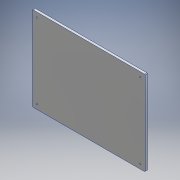
# Autodesk Inventor part: Breadboard
Saved by Autodesk Inventor 2016 (Build 200138000, 138)
## iProperties
Created: 2015-08-25
Part Number: Breadboard
Material: Aluminum 6061
Document SubType Name: Modeling
Designer: Conor Mow-Lowry
Density: 2.7 g/cm^3
Appearance: Aluminum - Flat
Author: Conor Mow-Lowry
Autodesk Inventor part; units mm, degrees
ref_plane "YZ Plane" through (0, 0, 0) normal (1, 0, 0) x (0, 1, 0)
ref_plane "XZ Plane" through (0, 0, 0) normal (0, 1, 0) x (-1, 0, 0)
ref_plane "XY Plane" through (0, 0, 0) normal (0, 0, 1) x (1, 0, 0)
sketch "Sketch1" plane through (0, 0, 0) normal (0, 1, 0) x (-1, 0, 0)
  line L0 (300, 225) -> (-300, 225)
  line L1 (-300, 225) -> (-300, -225)
  line L2 (-300, -225) -> (300, -225)
  line L3 (300, -225) -> (300, 225)
  line L4 (300, 225) -> (-300, -225) construction
  line L5 (-300, 225) -> (300, -225) construction
  point P0 (0, 0)
  dimension "d0" = 600
  dimension "d1" = 450
  constraints: 12 end point, 2 midpoint, 2 parallel, 1 horizontal, 1 perpendicular
  measures "d0" distance of L2.end L1.end
  measures "d1" distance of L1.end L0.end
extrude "Extrusion1" add sketch "Sketch1" along normal blind 12.7
fillet "Fillet1" radius 3 4 edges at (300, 6.35, 225) (300, 6.35, -225) (-300, 6.35, 225) (-300, 6.35, -225)
sketch "Sketch2" plane through (0, 12.7, 0) normal (0, 1, 0) x (1, 0, 0)
  line L0 (-300, 222) -> (-300, -222) projected
  line L1 (297, 225) -> (-297, 225) projected
  line L2 (-297, -225) -> (297, -225) projected
  line L3 (300, -222) -> (300, 222) projected
  line L4 (0, 225) -> (0, -225) construction
  line L5 (-300, 0) -> (300, 0) construction
  point P0 (0, 0)
  point P1 (-275, 200)
  point P2 (275, 200)
  point P3 (-275, -200)
  point P4 (275, -200)
  dimension "d5" = 25
  dimension "d6" = 25
  constraints: 4 end point, 4 midpoint, 3 symmetric about line
  measures "d5" distance from line of L1 point (-275, 200)
  measures "d6" distance from line of L0 point (-275, 200)
hole "Hole1" at (-275, 12.7, -200) at (275, 12.7, -200) at (275, 12.7, 200) at (-275, 12.7, 200) direction (0, -1, 0) diameter 6.6 end through all counterbore diameter 11 counterbore depth 6 clearance for "Socket Head Cap Screw" size "M6" standard "Ansi Metric M Profile"
body "Solid1"
